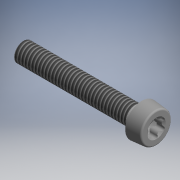
# Autodesk Inventor part: ISO 14580 M4x25
Saved by Autodesk Inventor 2017.3 (Build 213256000, 256)
## iProperties
Part Number: ISO 14580 M4x25
Material: Generic
Catalog Web Link: www.cadenas.de
Description: ISO-14580-Zylinderschrauben mit Innensechsrund, niedriger Kopf
Vendor: FESTO
Document SubType Name: Modeling
Designer: partserver
Manufacturer: FESTO
Mass: 0.401539 g
Surface Area: 4.72919 cm^2
Volume: 0.401539 cm^3
Density: 1 g/cm^3
Appearance: PSOLRGB-175-175-175
Category: PARTsolutions
Company: FESTO
Title: ISO 14580 M4x25
Author: Cadenas PARTsolutions
Comments: Zylinderschrauben mit Innensechsrund, niedriger Kopf
PSOL_IDENT_0: {$CADENAS_DATA\23d-libs\festo\zyl_zubeh\iso_14580\dineniso14580.prj},188 {VTYP=3D},{NB=ISO 14580 M4x
PSOL_IDENT_1: 25},{LINA=ISO 14580 M4x25},{NN=ISO-14580},{DATE=29.05.2015 09:58:39},{GEOMDATE=29.05.2015 09:58:27},
PSOL_IDENT_2: {VERSION=v080417071034},{LINEID=1010},{WBVAR=},{WBNUMERIC=}  {NB=ISO 14580 M4x25},{LINA=ISO 14580 M4
PSOL_IDENT_3: x25},{KT=DUMMY},{IDNR=},{D=4.000},{D3=3.141},{P=0.700},{L=25.000},{B=23.6},{X=1.750},{A1=1.400},{DK=
PSOL_IDENT_4: 7.000},{DA=4.700},{K=3.100},{R=0.200},{W=1.100},{NR=20},{A=3.950},{T=1.660},{NENN=M4x25},{V=1.000}
NB: ISO 14580 M4x25
NN: ISO-14580
NT: Zylinderschrauben mit Innensechsrund, niedriger Kopf
NBSYN: ISO 14580 $NENN.
LINA: ISO 14580 M4x25
CATALOG: Festo
ROWDESC: M4x25
D: 4
D3: 3.141
P: 0.7
L: 25
B: 23.6
X: 1.75
A1: 1.4
DK: 7
DA: 4.7
K: 3.1
R: 0.2
W: 1.1
NR: 20
A: 3.95
T: 1.66
SUPPLIER: FESTO
ARTICLENO: ISO 14580 M4x25
BOMINFO: ISO 14580 M4x25
CREATOR: CADENAS GmbH
Autodesk Inventor part; units mm, degrees
sketch "Skizze_2" plane through (-3.1, 0, 0) normal (1, 0, 0) x (0, 0, -1)
  arc A0 (-1.6711, 0.3843) -> (-1.6711, -0.3843) centre (-1.58, 0) ccw
  arc A1 (-1.1684, -1.2551) -> (-1.6711, -0.3843) centre (-1.8307, -1.0569) ccw
  arc A2 (-1.1684, -1.2551) -> (-0.5027, -1.6394) centre (-0.79, -1.3683) ccw
  arc A3 (0.5027, -1.6394) -> (-0.5027, -1.6394) centre (0, -2.1139) ccw
  arc A4 (0.5027, -1.6394) -> (1.1684, -1.2551) centre (0.79, -1.3683) ccw
  arc A5 (1.6711, -0.3843) -> (1.1684, -1.2551) centre (1.8307, -1.0569) ccw
  arc A6 (1.6711, -0.3843) -> (1.6711, 0.3843) centre (1.58, 0) ccw
  arc A7 (1.1684, 1.2551) -> (1.6711, 0.3843) centre (1.8307, 1.0569) ccw
  arc A8 (1.1684, 1.2551) -> (0.5027, 1.6394) centre (0.79, 1.3683) ccw
  arc A9 (-0.5027, 1.6394) -> (0.5027, 1.6394) centre (0, 2.1139) ccw
  arc A10 (-0.5027, 1.6394) -> (-1.1684, 1.2551) centre (-0.79, 1.3683) ccw
  arc A11 (-1.6711, 0.3843) -> (-1.1684, 1.2551) centre (-1.8307, 1.0569) ccw
  constraints: 24 point on circle, 12 centre point
sketch "Skizze_3" plane through (0, 0, 0) normal (0, 0, 1) x (1, 0, 0)
  line L0 (-0.1, 0) -> (-0.2997, 0)
  line L1 (-0.2997, 0) -> (-1.4977, 2.075)
  line L2 (-1.4977, 2.075) -> (-0.1, 2.075)
  line L3 (-0.1, 2.075) -> (-0.1, 0)
  line L4 (-0.1, 0) -> (-0.2997, 0)
  constraints: 10 end point
sketch "Skizze_5" plane through (0, 0, 0) normal (0, 0, 1) x (1, 0, 0)
  line L0 (25, 0) -> (-3.1, 0)
  line L1 (-3.1, 0) -> (-3.1, 3.2288)
  line L2 (-3.1, 3.2288) -> (0, 3.5)
  line L3 (0, 3.5) -> (0, 1.7853)
  line L4 (0, 1.7853) -> (1.028, 1.7853)
  line L5 (1.028, 1.7853) -> (1.4, 2)
  line L6 (1.4, 2) -> (25, 2)
  line L7 (25, 2) -> (25, 0)
  line L8 (25, 0) -> (-3.1, 0)
  constraints: 18 end point
revolve "Revolution1" add sketch "Skizze_5" angle 360 about axis through (25, 0, 0) along (1, 0, 0)
thread "Thread1" size "M4x0.7" class "6g" standard "ISO Metric profile" full length
sketch "Sketch_1" plane through (0, 0, 0) normal (0, 0, 1) x (1, 0, 0)
  line L0 (0.2, 0) -> (-0.1, 0)
  line L1 (-0.1, 1.6853) -> (0.2, 1.6853)
  line L2 (0.2, 1.6853) -> (0.2, 1.7853)
  arc A0 (0, 1.9852) -> (0.2, 1.7853) centre (0.2, 1.9853) ccw
  line L3 (0, 1.9852) -> (-0.1, 1.9852)
  line L4 (-0.1, 1.9852) -> (-0.1, 1.6853)
  constraints: 10 end point, 2 point on circle, 1 centre point
revolve "Revolution2" add sketch "Sketch_1" angle 360 about axis through (0.2, 0, 0) along (1, 0, 0)
sketch "Sketch_2" plane through (0, 0, 0) normal (0, 0, 1) x (1, 0, 0)
  line L0 (-1.9597, 0) -> (-3.1, 0)
  line L1 (-3.1, 0) -> (-3.1, 1.975)
  line L2 (-3.1, 1.975) -> (-1.9597, 0)
  line L3 (-1.9597, 0) -> (-3.1, 0)
  constraints: 8 end point
revolve "Revolution3" cut sketch "Sketch_2" angle 360 about axis through (-1.9597, 0, 0) along (1, 0, 0)
sketch "Sketch_3" plane through (0, 0, 0) normal (0, 0, 1) x (1, 0, 0)
  line L0 (50, 0) -> (-3.1, 0)
  line L1 (-3.6, 8.4) -> (-3.6, 2.9081)
  line L2 (-3.6, 2.9081) -> (-3.1, 2.9081)
  arc A0 (-2.7805, 3.2567) -> (-3.1, 2.9081) centre (-2.75, 2.9081) ccw
  line L3 (-2.7805, 3.2567) -> (-2.7805, 8.4)
  line L4 (-2.7805, 8.4) -> (-3.6, 8.4)
  constraints: 10 end point, 2 point on circle, 1 centre point
revolve "Revolution4" cut sketch "Sketch_3" angle 360 about axis through (50, 0, 0) along (1, 0, 0)
extrude "Extrusion1" cut sketch "Skizze_2" along normal blind 2.79
revolve "Revolution5" add sketch "Skizze_3" angle 360 about axis through (-0.1, 0, 0) along (1, 0, 0)
ref_plane "IP1_XY" through (0, 0, 0) normal (1, 0, 0) x (0, 0, -1)
ref_plane "IP1_YZ" through (0, 0, 0) normal (0, 0, -1) x (0, 1, 0)
ref_plane "IP1_ZX" through (0, 0, 0) normal (0, 1, 0) x (1, 0, 0)
body "Solid1"
